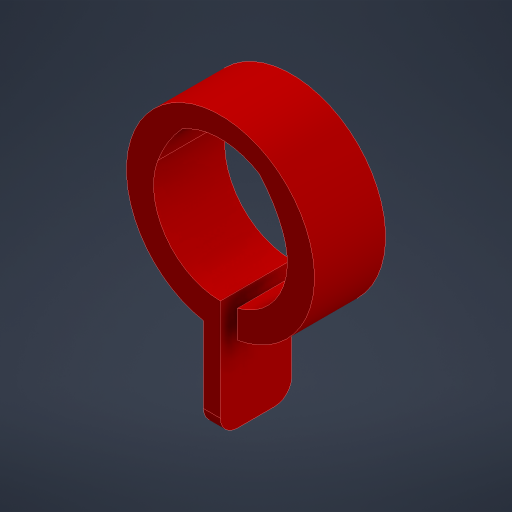
# Autodesk Inventor part: Laser Switch
Saved by Autodesk Inventor 2023.4 (Build 274418000, 418)
## iProperties
Created: 2024-05-15
Part Number: Laser Switch
Material: Generic
Document SubType Name: Modeling
Designer: xSibe
Density: 1 g/cm^3
Appearance: Plastic Dark Red
Author: xSibe
Autodesk Inventor part; units mm, degrees
ref_plane "YZ Plane" through (0, 0, 0) normal (1, 0, 0) x (0, 1, 0)
ref_plane "XZ Plane" through (0, 0, 0) normal (0, 1, 0) x (-1, 0, 0)
ref_plane "XY Plane" through (0, 0, 0) normal (0, 0, 1) x (1, 0, 0)
sketch "Sketch1" plane through (0, 0, 0) normal (0, 0, 1) x (1, 0, 0)
  circle A0 centre (0, 0) radius 9.875
  circle A1 centre (0, 0) radius 12.875
  line L0 (0, -9.875) -> (2.5, -9.875)
  line L1 (2.5, -9.875) -> (2.5, -19.875)
  line L2 (2.5, -19.875) -> (0, -19.875)
  line L3 (0, -19.875) -> (0, -9.875)
  line L4 (0, 0) -> (0, -9.875)
  line L5 (2.5, -9.875) -> (0, -9.875)
  line L6 (0, -9.875) -> (0, 0)
  line L7 (0, 0) -> (2.5, 0)
  line L8 (2.5, 0) -> (2.5, -9.875)
  line L9 (0, 9.875) -> (0, 12.875)
  line L10 (0, 12.875) -> (-1.25, 12.875)
  line L11 (-1.25, 12.875) -> (1.25, 12.875)
  line L12 (0, 9.875) -> (0, 0)
  line L13 (-1.25, 12.875) -> (-1.25, 12.8142)
  line L14 (1.25, 12.875) -> (1.25, 12.8142)
  arc A2 (-1.25, 12.8142) -> (-9.25, 3.4573) centre (7.5787, -2.8327) ccw
  arc A3 (9.25, 3.4573) -> (1.25, 12.8142) centre (-7.5787, -2.8327) ccw
  circle A4 centre (0, 0) radius 13.875
  line L15 (0, -9.875) -> (-2.5, -9.875)
  line L16 (-2.5, -9.875) -> (-2.5, -27.375)
  line L17 (-2.5, -27.375) -> (0, -27.375)
  line L18 (0, -27.375) -> (0, -9.875)
  line L19 (0, 0) -> (-9.25, 0)
  line L20 (-9.25, 0) -> (-9.25, 3.4573)
  line L21 (0, 0) -> (9.25, 0)
  line L22 (9.25, 0) -> (9.25, 3.4573)
  circle A5 centre (0, 0) radius 10.875
  line L23 (0, -9.875) -> (2.5, -9.875)
  line L24 (2.5, -9.875) -> (2.5, -27.375)
  line L25 (2.5, -27.375) -> (0, -27.375)
  line L26 (0, -27.375) -> (0, -9.875)
  point P0 (2.5, -9.5533)
  point P1 (2.5, -13.6479)
  point P2 (0, -13.875)
  point P3 (0, -19.875)
  point P4 (-2.5, -13.6479)
  point P5 (0, -12.875)
  point P6 (2.5, -12.6299)
  point P7 (0, 12.875)
  point P8 (5.7151, 9.2522)
  point P9 (-5.7151, 9.2522)
  point P10 (0, -27.375)
  point P11 (2.5, -19.875)
  dimension "d0" = 19.75
  dimension "d1" = 3
  dimension "d3" = 2.5
  dimension "d4" = 10
  dimension "d5" = 1.25
  dimension "d6" = 2.5
  dimension "d7" = 1
  dimension "d14" = 2.5
  dimension "d15" = 17.5
  dimension "d16" = 9.25
  dimension "d17" = 9.25
  dimension "d19" = 1
  dimension "d22" = 2.5
  dimension "d23" = 17.5
  constraints: 54 end point, 11 point on circle, 9 parallel, 7 perpendicular, 6 centre point, 6 horizontal, 3 vertical, 2 tangent, 1 coincident, 1 collinear, 1 point on line
  measures "d0" diameter of A0
  measures "d1" radial gap between concentric circles of A0 A1
  measures "d3" distance of L1.end L2.end
  measures "d4" distance of L0.end L1.end
  measures "d5" distance of L9.end L10.end
  measures "d6" distance of L10.end L11.end
  measures "d7" radial gap between concentric circles of A1 A4
  measures "d14" distance of L17.end L16.end
  measures "d15" distance of L16.end L15.end
  measures "d16" distance of L4.start L19.end
  measures "d17" distance of L4.start L21.end
  measures "d19" radial gap between concentric circles of A0 A5
  measures "d22" distance of L24.end L25.end
  measures "d23" distance of L23.end L24.end
extrude "Extrusion1" add sketch "Sketch1" along normal blind 2.5 contours A0 A3 A5 L1 L8 | A0 L9 A5 A3 | L8 L0 A0 | A0 A2 A5 L9 | A5 L9 A1 A3 | A3 A1 L1 A5 | L15 L16 A5 A2 A0 | L0 L1 A5 L3 | L3 A5 L16 L15 | A5 A2 A1 L9 | L14 L11 L10 L13 A1 L16 A4 L1 | A1 L11 L14 | A5 L1 A1 L3 | L3 A1 L16 A5 | A5 L16 A1 A2 | A1 L13 L10 | L3 A4 L16 A1 | A1 L1 A4 L3 | A4 L1 L2 L3 | L3 L18 L17 L16 A4 | L2 L24 L25 L18
extrude "Extrusion2" add sketch "Sketch1" along normal blind 5.5 from surface at 2.5 contours A0 A3 A5 L1 L8 | L8 L0 A0 | A3 A1 L1 A5 | L15 L16 A5 A2 A0 | L0 L1 A5 L3 | L3 A5 L16 L15 | L14 L11 L10 L13 A1 L16 A4 L1 | A1 L11 L14 | A5 L1 A1 L3 | L3 A1 L16 A5 | A5 L16 A1 A2 | A1 L13 L10 | L3 A4 L16 A1 | A1 L1 A4 L3 | A4 L1 L2 L3 | L3 L18 L17 L16 A4 | L2 L24 L25 L18
extrude "Extrusion3" add sketch "Sketch1" along normal blind 2.5 from surface at 8 contours A0 A3 A5 L1 L8 | A0 L9 A5 A3 | L8 L0 A0 | A0 A2 A5 L9 | A5 L9 A1 A3 | A3 A1 L1 A5 | L15 L16 A5 A2 A0 | L0 L1 A5 L3 | L3 A5 L16 L15 | A5 A2 A1 L9 | L14 L11 L10 L13 A1 L16 A4 L1 | A1 L11 L14 | A5 L1 A1 L3 | L3 A1 L16 A5 | A5 L16 A1 A2 | A1 L13 L10 | L3 A4 L16 A1 | A1 L1 A4 L3 | A4 L1 L2 L3 | L3 L18 L17 L16 A4 | L2 L24 L25 L18
fillet "Fillet1" radius 2.5 2 edges at (-1.25, 12.8142, 5.25) (1.25, 12.8142, 5.25)
extrude "Extrusion4" cut sketch "Sketch1" against normal up to surface (2.5 mm away) from surface at 10.5 contours A0 L9 A5 A3 | A0 A2 A5 L9
extrude "Extrusion5" cut sketch "Sketch1" along normal up to surface (10.5 mm away) from surface at 0 contours L8 L0 A0 | L0 L1 A5 L3 | A5 L1 A1 L3 | A1 L1 A4 L3 | A4 L1 L2 L3 | L2 L24 L25 L18
fillet "Fillet2" radius 2.5 2 edges at (-1.25, -27.375, 10.5) (-1.25, -27.375, 0)
body "Solid1"
